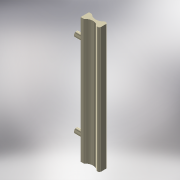
# Autodesk Inventor part: manija
Saved by Autodesk Inventor 2016 (Build 200138000, 138)
## iProperties
Created: 2014-06-15
Part Number: manija
Material: Genérico
Document SubType Name: Modeling
Designer: Mecatronica
Density: 1 g/cm^3
Appearance: Nickel
Author: Mecatronica
Autodesk Inventor part; units mm, degrees
ref_plane "YZ Plane" through (0, 0, 0) normal (1, 0, 0) x (0, 1, 0)
ref_plane "XZ Plane" through (0, 0, 0) normal (0, 1, 0) x (-1, 0, 0)
ref_plane "XY Plane" through (0, 0, 0) normal (0, 0, 1) x (1, 0, 0)
sketch "Boceto1" plane through (0, 0, 0) normal (0, 0, 1) x (1, 0, 0)
  arc A0 (786.2416, 528.0882) -> (772.0751, 528.0882) centre (779.1584, 521.0294) ccw
  arc A1 (786.2416, 528.0882) -> (772.0751, 528.0882) centre (779.1584, 521.0294) ccw
  line L0 (767.7, 527.5) -> (770.6584, 527.5)
  line L1 (767.7, 527.5) -> (770.6584, 527.5)
  arc A2 (790.2, 535.5) -> (788.2, 537.5) centre (788.2, 535.5) ccw
  line L2 (787.6583, 537.5) -> (788.2, 537.5)
  line L3 (787.6583, 537.5) -> (788.2, 537.5)
  arc A3 (787.6583, 537.5) -> (786.2416, 536.9118) centre (787.6583, 535.5) ccw
  arc A4 (787.6583, 537.5) -> (786.2416, 536.9118) centre (787.6583, 535.5) ccw
  arc A5 (772.0751, 536.9118) -> (786.2416, 536.9118) centre (779.1584, 543.9706) ccw
  arc A6 (772.0751, 536.9118) -> (786.2416, 536.9118) centre (779.1584, 543.9706) ccw
  line L4 (790.2, 535.5) -> (790.2, 532.5)
  arc A7 (786.2416, 528.0882) -> (787.6583, 527.5) centre (787.6583, 529.5) ccw
  arc A8 (786.2416, 528.0882) -> (787.6583, 527.5) centre (787.6583, 529.5) ccw
  line L5 (787.6583, 527.5) -> (788.2, 527.5)
  line L6 (787.6583, 527.5) -> (788.2, 527.5)
  arc A9 (788.2, 527.5) -> (790.2, 529.5) centre (788.2, 529.5) ccw
  line L7 (790.2, 529.5) -> (790.2, 532.5)
  line L8 (790.2, 529.5) -> (790.2, 532.5)
  arc A10 (788.2, 527.5) -> (790.2, 529.5) centre (788.2, 529.5) ccw
  line L9 (767.7, 537.5) -> (770.6584, 537.5)
  arc A11 (772.0751, 536.9118) -> (770.6584, 537.5) centre (770.6584, 535.5) ccw
  arc A12 (772.0751, 536.9118) -> (770.6584, 537.5) centre (770.6584, 535.5) ccw
  line L10 (767.7, 537.5) -> (770.6584, 537.5)
  line L11 (767.7, 532.5) -> (767.7, 537.5)
  line L12 (767.7, 532.5) -> (767.7, 537.5)
  arc A13 (770.6584, 527.5) -> (772.0751, 528.0882) centre (770.6584, 529.5) ccw
  arc A14 (770.6584, 527.5) -> (772.0751, 528.0882) centre (770.6584, 529.5) ccw
  line L13 (767.7, 532.5) -> (767.7, 527.5)
  line L14 (767.7, 532.5) -> (767.7, 527.5)
  arc A15 (772.0751, 536.9118) -> (786.2416, 536.9118) centre (779.1584, 543.9706) ccw
  line L15 (787.6583, 537.5) -> (788.2, 537.5)
  line L16 (767.7, 537.5) -> (770.6584, 537.5)
  arc A16 (787.6583, 537.5) -> (786.2416, 536.9118) centre (787.6583, 535.5) ccw
  arc A17 (772.0751, 536.9118) -> (770.6584, 537.5) centre (770.6584, 535.5) ccw
  arc A18 (790.2, 535.5) -> (788.2, 537.5) centre (788.2, 535.5) ccw
  line L17 (767.7, 532.5) -> (767.7, 537.5)
  line L18 (790.2, 535.5) -> (790.2, 532.5)
  point P0 (790.2, 537.5)
  point P1 (790.2, 537.5)
  point P2 (786.7828, 537.5)
  point P3 (786.7828, 537.5)
  point P4 (786.7828, 527.5)
  point P5 (786.7828, 527.5)
  point P6 (790.2, 527.5)
  point P7 (790.2, 527.5)
  point P8 (771.534, 537.5)
  point P9 (771.534, 537.5)
  point P10 (771.534, 527.5)
  point P11 (771.534, 527.5)
  point P12 (779.1584, 533.9706)
  point P13 (771.534, 537.5)
  point P14 (790.2, 537.5)
  point P15 (786.7828, 537.5)
  constraints: 48 point on circle, 38 end point, 19 centre point, 19 point on line
extrude "Extrusión1" add sketch "Boceto1" along normal blind 150
sketch "Sketch3" plane through (767.7, 527.5, 0) normal (-1, 0, 0) x (0, 0, 1)
  line L0 (0, 10) -> (0, 0) construction
  line L1 (0, 0) -> (150, 0) construction
  line L2 (150, 10) -> (150, 0) construction
  line L3 (0, 10) -> (150, 10) construction
  line L4 (0, 2) -> (0, 8) projected
  line L5 (0, 5) -> (150, 5) construction
  line L6 (150, 2) -> (150, 8) projected
  circle A0 centre (25, 5) radius 3
  line L7 (0, 0) -> (150, 0) projected
  line L8 (75, 0) -> (75, 10) construction
  line L9 (0, 10) -> (150, 10) projected
  circle A1 centre (125, 5) radius 3
  point P0 (0, -527.5)
  dimension "d6" = 6
  dimension "d7" = 50
  constraints: 4 end point, 4 midpoint, 2 centre point, 1 point on line, 1 symmetric about line, 1 other
  measures "d6" diameter of A0
  measures "d7" distance from line of L8 A0.centre
extrude "Extrusion3" add sketch "Sketch3" along normal blind 10
